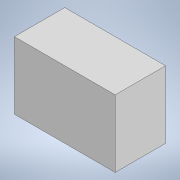
# Autodesk Inventor part: aircraft03_02
Saved by Autodesk Inventor 2022 (Build 260153000, 153)
## iProperties
Created: 2024-05-29
Part Number: aircraft03_02
Material: 一般
Document SubType Name: Modeling
Designer: numer
Density: 1 g/cm^3
Appearance: 既定
Author: numer
Autodesk Inventor part; units mm, degrees
ref_plane "YZ Plane" through (0, 0, 0) normal (1, 0, 0) x (0, 1, 0)
ref_plane "XZ Plane" through (0, 0, 0) normal (0, 1, 0) x (-1, 0, 0)
ref_plane "XY Plane" through (0, 0, 0) normal (0, 0, 1) x (1, 0, 0)
sketch "スケッチ1" plane through (0, 0, 0) normal (0, 1, 0) x (-1, 0, 0)
  line L0 (1000, 1500) -> (-5000, 1500)
  line L1 (-5000, 1500) -> (-5000, -1500)
  line L2 (-5000, -1500) -> (1000, -1500)
  line L3 (1000, -1500) -> (1000, 1500)
  line L4 (2200, 0) -> (-6200, 0) projected
  line L5 (0, -2100) -> (0, 2100) projected
  point P0 (0, 0)
  dimension "d0" = 3000
  dimension "d1" = 1000
  dimension "d2" = 6000
  constraints: 8 end point, 2 parallel, 1 horizontal, 1 perpendicular, 1 other
  measures "d0" distance of L2.end L0.start
  measures "d1" distance between parallel lines of L3 L5
  measures "d2" distance of L0.start L0.end
extrude "押し出し1" add sketch "スケッチ1" along normal mid plane 4000
